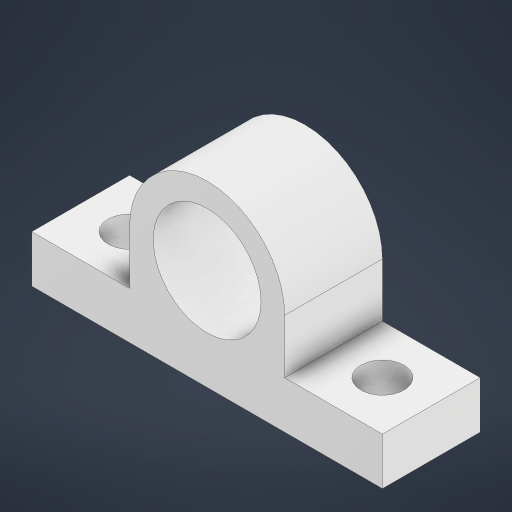
# Autodesk Inventor part: Mauch_Power_Button_Bracket
Saved by Autodesk Inventor 2024.1 (Build 281209000, 209)
## iProperties
Created: 2023-11-30
Part Number: Mauch_Power_Button_Bracket
Material: ABS Plastic
Document SubType Name: Modeling
Designer: dzw04
Density: 1.06 g/cm^3
Appearance: Smooth - White
Author: dzw04
Autodesk Inventor part; units mm, degrees
ref_plane "YZ Plane" through (0, 0, 0) normal (1, 0, 0) x (0, 1, 0)
ref_plane "XZ Plane" through (0, 0, 0) normal (0, 1, 0) x (-1, 0, 0)
ref_plane "XY Plane" through (0, 0, 0) normal (0, 0, 1) x (1, 0, 0)
sketch "Sketch1" plane through (0, 0, 0) normal (0, 0, 1) x (1, 0, 0)
  line L0 (-13, -1.75) -> (13, -1.75)
  line L1 (13, -1.75) -> (13, 1.75)
  line L2 (13, 1.75) -> (-13, 1.75)
  line L3 (-13, 1.75) -> (-13, -1.75)
  line L4 (-13, -1.75) -> (13, 1.75) construction
  line L5 (13, -1.75) -> (-13, 1.75) construction
  line L6 (0, 1.75) -> (0, 5.75)
  circle A0 centre (0, 5.75) radius 4
  circle A1 centre (0, 5.75) radius 5.75
  line L7 (-5.75, 5.75) -> (-5.75, 1.75)
  line L8 (5.75, 5.75) -> (5.75, 1.75)
  point P0 (0, 0)
  dimension "d0" = 26
  dimension "d1" = 3.5
  dimension "d2" = 4
  dimension "d3" = 8
  dimension "d4" = 11.5
  constraints: 18 end point, 3 midpoint, 3 perpendicular, 2 centre point, 2 coincident, 2 parallel, 2 point on circle, 2 point on line, 1 horizontal, 1 vertical
  measures "d0" distance of L2.end L1.end
  measures "d1" distance of L1.end L0.end
  measures "d2" distance of L6.start L6.end
  measures "d3" diameter of A0
  measures "d4" diameter of A1
extrude "Extrusion1" add sketch "Sketch1" along normal blind 7.25
sketch "Sketch2" plane through (-13, -1.75, 0) normal (0, -1, 0) x (1, 0, 0)
  line L0 (13, 0) -> (13, 7.25)
  line L1 (9, 7.25) -> (17, 7.25) projected
  line L2 (13, 3.625) -> (22.375, 3.625)
  line L3 (22.375, 3.625) -> (3.625, 3.625)
  circle A0 centre (22.375, 3.625) radius 1.6
  circle A1 centre (3.625, 3.625) radius 1.6
  dimension "d7" = 9.375
  dimension "d8" = 18.75
  dimension "d9" = 3.2
  dimension "d10" = 3.2
  constraints: 6 end point, 2 centre point, 2 coincident, 2 midpoint, 1 horizontal, 1 point on line
  measures "d7" distance of L2.start L2.end
  measures "d8" distance of L2.end L3.end
  measures "d9" diameter of A0
  measures "d10" diameter of A1
extrude "Extrusion2" cut sketch "Sketch2" against normal blind 7.25
body "Solid1"
